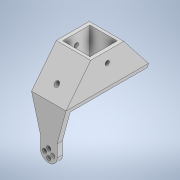
# Autodesk Inventor part: OutPut_Shaft_From_Gearbox
Saved by Autodesk Inventor 2022 (Build 260153000, 153)
## iProperties
Created: 2022-01-20
Part Number: OutPut_Shaft_From_Gearbox
Material: Generic
Document SubType Name: Modeling
Designer: Mlees
Density: 1 g/cm^3
Appearance: Default
Author: Mlees
Autodesk Inventor part; units mm, degrees
ref_plane "YZ Plane" through (0, 0, 0) normal (1, 0, 0) x (0, 1, 0)
ref_plane "XZ Plane" through (0, 0, 0) normal (0, 1, 0) x (-1, 0, 0)
ref_plane "XY Plane" through (0, 0, 0) normal (0, 0, 1) x (1, 0, 0)
sketch "Sketch1" plane through (0, 0, 0) normal (0, 0, 1) x (1, 0, 0)
  circle A0 centre (0, 4) radius 2
  circle A1 centre (-4, 0) radius 2
  circle A2 centre (0, -4) radius 2
  circle A3 centre (4, 0) radius 2
  line L0 (8, 11.7321) -> (15.5744, 40)
  line L1 (7, 8) -> (40.1288, 8) construction
  line L2 (-8, 11.7321) -> (-15.5744, 40)
  line L3 (8, 0) -> (8, 11.7321)
  line L4 (-8, 0) -> (-8, 11.7321)
  arc A4 (-8, 0) -> (8, 0) centre (0, 0) ccw
  line L5 (0, 43) -> (16.3782, 43)
  line L6 (16.3782, 43) -> (15.5744, 40)
  line L7 (-15.5744, 40) -> (-16.3782, 43)
  line L8 (-16.3782, 43) -> (0, 43)
  dimension "d2" = 4
  dimension "d5" = 360
  constraints: 18 end point, 5 centre point, 2 point on circle, 1 collinear, 1 horizontal, 1 point on line, 9 other
  measures "d2" diameter of A0
extrude "Extrusion1" add sketch "Sketch1" along normal blind 5
sketch "Sketch2" plane through (0, 0, 0) normal (0, 0, -1) x (-1, 0, 0)
  circle A0 centre (0, 0) radius 6.625
  dimension "d18" = 13.25
  constraints: 1 centre point, 1 coincident
  measures "d18" diameter of A0
extrude "Extrusion2" cut sketch "Sketch2" against normal blind 2
sketch "Sketch4" plane through (0, 0, 0) normal (0, 0, -1) x (-1, 0, 0)
  line L0 (-8, 11.7321) -> (-16.3782, 43) projected
  line L1 (-16.3782, 43) -> (16.3782, 43) projected
  line L2 (-16.3782, 43) -> (16.3782, 43)
  line L3 (0, 39.136) -> (15.3429, 39.136)
  line L4 (16.3782, 43) -> (8, 11.7321) projected
  line L5 (15.3429, 39.136) -> (16.3782, 43)
  line L6 (0, 39.136) -> (-15.3429, 39.136)
  line L7 (-15.3429, 39.136) -> (-16.3782, 43)
  point P0 (0, 0)
  constraints: 10 end point, 3 collinear, 2 point on line, 1 horizontal
extrude "Extrusion4" add sketch "Sketch4" along normal blind 73.5
sketch "Sketch5" plane through (-16.3782, 43, 5) normal (0, 1, 0) x (1, 0, 0)
  line L0 (0, 78.5) -> (32.7564, 78.5) projected
  line L1 (32.7564, 0) -> (0, 0) projected
  line L2 (0, 78.5) -> (32.7564, 78.5)
  line L3 (32.7564, 78.5) -> (32.7564, 0)
  line L4 (32.7564, 0) -> (0, 0)
  line L5 (0, 0) -> (0, 78.5)
  point P0 (16.3782, 5)
  constraints: 8 end point, 2 parallel, 1 horizontal, 1 perpendicular
extrude "Extrusion5" add sketch "Sketch5" along normal blind 30
sketch "Sketch6" plane through (16.3782, 43, -73.5) normal (1, 0, 0) x (0, 0, -1)
  line L0 (-78.5, 30) -> (0, 30) projected
  line L1 (-39.25, 30) -> (-26.55, 30)
  line L2 (-39.25, 30) -> (-51.95, 30)
  line L3 (-51.95, 30) -> (-54.95, 30)
  line L4 (-26.55, 30) -> (-23.55, 30)
  line L5 (0, -3.864) -> (0, 0) projected
  line L6 (-23.55, 30) -> (0, 0)
  line L7 (0, 0) -> (0, 30) projected
  line L8 (0, 0) -> (0, 30)
  line L9 (0, 30) -> (-23.55, 30)
  line L10 (-54.95, 30) -> (-78.5, 30)
  line L11 (-78.5, 0) -> (-78.5, 30) projected
  line L12 (-78.5, 30) -> (-78.5, 0)
  line L13 (-78.5, 0) -> (-54.95, 30)
  point P0 (-73.5, -43)
  dimension "d30" = 12.7
  dimension "d31" = 12.7
  dimension "d32" = 3
  dimension "d33" = 3
  constraints: 20 end point, 4 point on line, 3 collinear, 1 midpoint, 1 perpendicular
  measures "d30" distance of L1.start L1.end
  measures "d31" distance of L1.start L2.end
  measures "d32" distance of L2.end L3.end
  measures "d33" distance of L1.end L4.end
extrude "Extrusion6" cut sketch "Sketch6" against normal up to surface (32.7564 mm away)
sketch "Sketch7" plane through (-16.3782, 73, 5) normal (0, 1, 0) x (1, 0, 0)
  line L0 (0, 78.5) -> (0, 0) projected
  line L1 (0, 23.55) -> (32.7564, 23.55) projected
  line L2 (16.3782, 52.25) -> (3.3782, 52.25)
  line L3 (3.3782, 52.25) -> (3.3782, 26.25)
  line L4 (3.3782, 26.25) -> (29.3782, 26.25)
  line L5 (29.3782, 26.25) -> (29.3782, 52.25)
  line L6 (29.3782, 52.25) -> (16.3782, 52.25)
  point P0 (16.3782, 5)
  dimension "d37" = 13
  dimension "d38" = 26
  dimension "d39" = 26
  constraints: 10 end point, 4 perpendicular, 1 point on line
  measures "d37" distance of L2.start L2.end
  measures "d38" distance of L2.end L3.end
  measures "d39" distance of L3.end L4.end
extrude "Extrusion7" cut sketch "Sketch7" against normal blind 25.4
ref_plane "Work Plane1" through (0, 0, 2.5) normal (0, 0, 1) x (1, 0, 0)
sketch "Sketch8" plane through (0, 0, 2.5) normal (0, 0, 1) x (1, 0, 0)
  line L0 (16.3782, 43) -> (-16.3782, 43) projected
  circle A0 centre (0, 53) radius 2
  point P0 (0, 0)
  dimension "d43" = 4
  constraints: 1 centre point
  measures "d43" diameter of A0
extrude "Extrusion8" cut sketch "Sketch8" against normal through all
sketch "Sketch9" plane through (16.3782, 43, 5) normal (1, 0, 0) x (0, 0, -1)
  line L0 (26.25, 30) -> (52.25, 30) projected
  circle A0 centre (39.25, 20) radius 2
  point P0 (5, -43)
  dimension "d47" = 4
  constraints: 1 centre point
  measures "d47" diameter of A0
extrude "Extrusion9" cut sketch "Sketch9" against normal up to surface (32.7564 mm away)
body "Solid1"
